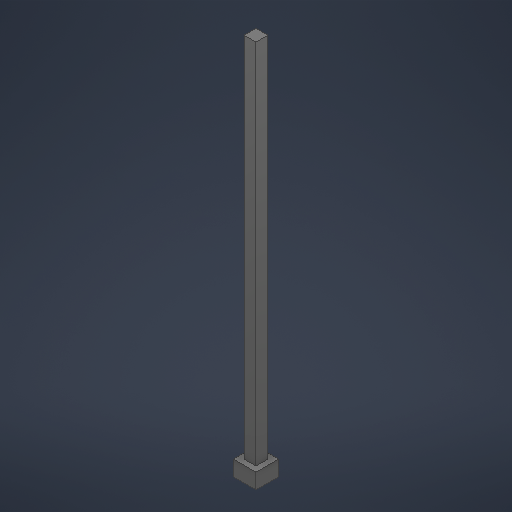
# Autodesk Inventor part: podstawa_rod
Saved by Autodesk Inventor 2027 (Build 310192060, 192F)
## iProperties
Created: 2026-08-24
Part Number: podstawa_rod
Material: Ogólny
Document SubType Name: Modeling
Designer: User
Density: 1 g/cm^3
Appearance: Domyślna
Author: User
Autodesk Inventor part; units mm, degrees
ref_plane "YZ Plane" through (0, 0, 0) normal (1, 0, 0) x (0, 1, 0)
ref_plane "XZ Plane" through (0, 0, 0) normal (0, 1, 0) x (-1, 0, 0)
ref_plane "XY Plane" through (0, 0, 0) normal (0, 0, 1) x (1, 0, 0)
sketch "Szkic1" plane through (0, 0, 0) normal (0, 1, 0) x (-1, 0, 0)
  line L0 (-7.4, 7.4) -> (7.4, 7.4)
  line L1 (7.4, 7.4) -> (7.4, -7.4)
  line L2 (7.4, -7.4) -> (-7.4, -7.4)
  line L3 (-7.4, -7.4) -> (-7.4, 7.4)
  line L4 (-7.4, 7.4) -> (7.4, -7.4) construction
  line L5 (7.4, 7.4) -> (-7.4, -7.4) construction
  line L6 (3.9, 3.9) -> (-3.9, 3.9)
  line L7 (-3.9, 3.9) -> (-3.9, -3.9)
  line L8 (-3.9, -3.9) -> (3.9, -3.9)
  line L9 (3.9, -3.9) -> (3.9, 3.9)
  line L10 (3.9, 3.9) -> (-3.9, -3.9) construction
  line L11 (-3.9, 3.9) -> (3.9, -3.9) construction
  point P0 (0, 0)
  dimension "d0" = 14.8
  dimension "d1" = 14.8
  dimension "d7" = 7.8
  dimension "d8" = 7.8
  constraints: 24 end point, 4 midpoint, 4 parallel, 2 horizontal, 2 perpendicular
  measures "d0" distance of L1.end L2.end
  measures "d1" distance of L0.end L1.end
  measures "d7" distance of L8.end L7.end
  measures "d8" distance of L7.end L6.end
extrude "Wyciągnięcie proste1" add sketch "Szkic1" against normal blind 10 contours L0 L1 L2 L3 | L9 L8 L7 L6
extrude "Wyciągnięcie proste2" add sketch "Szkic1" along normal blind 240 contours L9 L8 L7 L6
